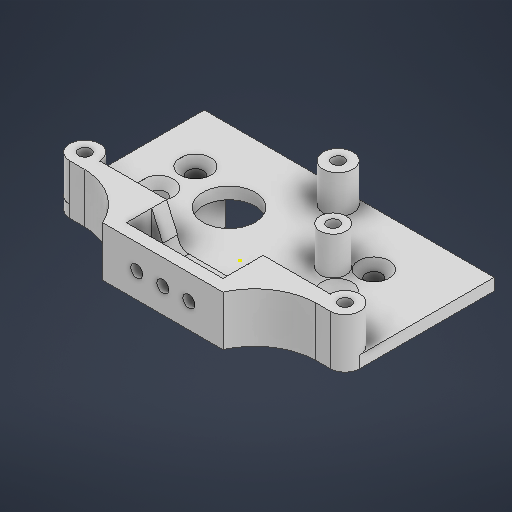
# Autodesk Inventor part: ПЕРЕДНИЙ ЗАХВАТ
Saved by Autodesk Inventor 2025 (Build 290162000, 162)
## iProperties
Created: 2025-02-17
Part Number: ПЕРЕДНИЙ ЗАХВАТ
Material: Типовые
Document SubType Name: Modeling
Designer: Phantom
Density: 1 g/cm^3
Appearance: По умолчанию
Author: Phantom
Autodesk Inventor part; units mm, degrees
ref_plane "YZ Plane" through (0, 0, 0) normal (1, 0, 0) x (0, 1, 0)
ref_plane "XZ Plane" through (0, 0, 0) normal (0, 1, 0) x (-1, 0, 0)
ref_plane "XY Plane" through (0, 0, 0) normal (0, 0, 1) x (1, 0, 0)
sketch "Эскиз1" plane through (0, 0, 0) normal (0, 1, 0) x (-1, 0, 0)
  line L0 (-30, 30.5) -> (30, 30.5)
  line L1 (30, 30.5) -> (30, -30.5)
  line L2 (30, -30.5) -> (-30, -30.5)
  line L3 (-30, -30.5) -> (-30, 30.5)
  line L4 (-30, 30.5) -> (30, 30.5) construction
  circle A0 centre (0, -26.5) radius 1.6
  circle A1 centre (-14, -11.15) radius 2.1
  circle A2 centre (14, -11.15) radius 7
  point P0 (0, 0)
  dimension "d0" = 60
  dimension "d2" = 61
  dimension "d3" = 30
  dimension "d4" = 3.2
  dimension "d5" = 4
  dimension "d6" = 4.2
  dimension "d7" = 19.35
  dimension "d8" = 28
  dimension "d9" = 14
  dimension "d11" = 19.35
  dimension "d13" = 16
  constraints: 10 end point, 3 centre point, 2 horizontal, 2 parallel, 1 collinear, 1 perpendicular
  measures "d0" distance of L0.start L0.end
  measures "d2" distance of L0.end L1.end
  measures "d3" distance from line of L3 A0.centre
  measures "d4" diameter of A0
  measures "d5" distance from line of L2 A0.centre
  measures "d6" diameter of A1
  measures "d7" distance from line of L2 A1.centre
  measures "d8" distance of A1.centre A2.centre
  measures "d9" diameter of A2
  measures "d11" distance from line of L2 A2.centre
  measures "d13" distance from line of L3 A1.centre
extrude "Выдавливание1" add sketch "Эскиз1" along normal blind 3.2
sketch "Эскиз2" plane through (0, 3.2, 0) normal (0, 1, 0) x (1, 0, 0)
  line L0 (30, 30.5) -> (-30, 30.5) projected
  line L1 (-30, 30.5) -> (-30, -5.65)
  line L2 (-30, 30.5) -> (-30, -30.5) projected
  line L3 (-30, -5.65) -> (30, -5.65)
  line L4 (-30, -5.65) -> (30, -5.65)
  line L5 (30, -5.65) -> (30, -9.65)
  line L6 (30, -9.65) -> (-30, -9.65)
  line L7 (-30, -9.65) -> (-30, -5.65)
  circle A0 centre (0, 26.5) radius 1.6 projected
  circle A1 centre (0, 26.5) radius 4
  line L8 (4, 26.5) -> (4, 30.5)
  line L9 (-4, 26.5) -> (-4, 30.5)
  point P0 (0, 0)
  dimension "d16" = 36.15
  dimension "d17" = 60
  dimension "d18" = 4
  dimension "d19" = 8
  constraints: 16 end point, 4 perpendicular, 3 point on line, 2 parallel, 2 point on circle, 2 tangent, 1 centre point, 1 coincident, 1 horizontal
  measures "d16" distance of L0.end L1.end
  measures "d17" distance of L5.end L6.end
  measures "d18" distance of L4.end L5.end
  measures "d19" diameter of A1
extrude "Выдавливание2" add sketch "Эскиз2" along normal blind 10.2 contours A1 | L3 L5 L6 L2
sketch "Эскиз3" plane through (0, 0, 0) normal (0, -1, 0) x (1, 0, 0)
  arc A0 (-23.679, -20.65) -> (-23.512, -21.65) centre (-22.7453, -21.008) ccw
  line L0 (-24.037, -20.65) -> (-24.037, -1.65)
  arc A1 (-23.512, -0.65) -> (-23.679, -1.65) centre (-22.7453, -1.292) ccw
  line L1 (17.25, -0.65) -> (-22.25, -0.65)
  arc A2 (16.988, -1.65) -> (15.988, -0.65) centre (15.988, -1.65) ccw
  line L2 (15.963, -20.65) -> (15.963, -1.65)
  arc A3 (15.988, -21.65) -> (16.988, -20.65) centre (15.988, -20.65) ccw
  line L3 (17.25, -21.65) -> (-22.25, -21.65)
  circle A4 centre (-28.037, -16.15) radius 2.1
  circle A5 centre (-28.037, -6.15) radius 2.1
  circle A6 centre (19.963, -6.15) radius 2.1
  circle A7 centre (19.963, -16.15) radius 2.1
  line L4 (2.4, 0.15) -> (9.6, 0.15)
  circle A8 centre (-14, -11.15) radius 7 projected
  line L5 (-28.037, -2.15) -> (-24.037, -2.15)
  line L6 (-28.037, -2.15) -> (-32.037, -2.15)
  line L7 (-32.037, -2.15) -> (-32.037, -20.15)
  line L8 (-32.037, -20.15) -> (-24.037, -20.15)
  line L9 (-2.5, -0.65) -> (-2.5, -38)
  line L10 (19.963, -2.15) -> (15.963, -2.15)
  line L11 (19.963, -2.15) -> (23.963, -2.15)
  line L12 (23.963, -2.15) -> (23.963, -20.15)
  line L13 (23.963, -20.15) -> (15.963, -20.15)
  line L14 (16.988, -20.65) -> (16.988, -20.15)
  line L15 (17.704, -2.15) -> (16.988, -1.65)
  line L16 (-30, -30.5) -> (-30, 30.5) projected
  point P0 (0, 0)
  point P1 (-14, -11.15)
  point P2 (24.738, -11.15)
  point P3 (-28.037, -6.15)
  point P4 (19.846, -6.15)
  point P5 (-28.037, -6.15)
  constraints: 32 end point, 8 centre point, 8 point on circle, 4 point on line, 2 perpendicular, 2 vertical, 1 coincident, 1 midpoint
extrude "Выдавливание3" add sketch "Эскиз3" along normal blind 11 contours L8 L16 A4 A5 L6 L5 L0 | L8 L7 L6 L16 A5 A4 | L10 L11 L12 L13 L2
sketch "Эскиз4" plane through (0, 0, 0) normal (0, 1, 0) x (1, 0, 0)
  line L0 (-30, 5.4039) -> (-30, 2.15) projected
  line L1 (-32.037, 20.15) -> (-30, 20.15) projected
  line L2 (-32.037, 2.15) -> (-32.037, 20.15) projected
  line L3 (-30, 2.15) -> (-32.037, 2.15) projected
  line L4 (30, -9.65) -> (-30, -9.65) projected
  line L5 (-30, -9.65) -> (-30, -30.5) projected
  line L6 (-30, -30.5) -> (30, -30.5) projected
  line L7 (30, -30.5) -> (30, -9.65) projected
  line L8 (-30, -30.5) -> (-31.25, -30.5)
  line L9 (-31.25, -30.5) -> (-31.25, 30.5)
  line L10 (-31.25, 30.5) -> (-30, 30.5)
  line L11 (-30, 30.5) -> (-30, -30.5)
  line L12 (30, 30.5) -> (-30, 30.5) projected
  line L13 (-30, 15.4039) -> (-30, 6.8961) projected
  arc A0 (-30, 16.8961) -> (-30, 15.4039) centre (-28.037, 16.15) ccw projected
  line L14 (-30, 20.15) -> (-30, 16.8961) projected
  arc A1 (-30, 6.8961) -> (-30, 5.4039) centre (-28.037, 6.15) ccw projected
  point P0 (0, 0)
  point P1 (-31.25, 20.15)
  point P2 (-31.25, 2.15)
  point P3 (-30, 2.15)
  point P4 (-30, 5.4039)
  point P5 (-30, 2.15)
  point P6 (-31.25, 2.15)
  point P7 (-31.25, 20.15)
  dimension "d25" = 0
  constraints: 8 end point, 2 parallel, 1 collinear, 1 horizontal, 1 perpendicular
  measures "d25" distance between parallel lines of L10 L12
extrude "Выдавливание4" add sketch "Эскиз4" along normal up to surface (3.2 mm away) contours A1 L11 | L0 L3 L9 L1 L11 A0 A1 | L11 L5 L8 L9 L3 | A0 L11 | L9 L10 L11 L1
sketch "Эскиз5" plane through (0, 3.2, 0) normal (0, 1, 0) x (1, 0, 0)
  circle A0 centre (14, 11.15) radius 2.1 projected
  circle A1 centre (-14, 11.15) radius 7 projected
  circle A2 centre (0, 26.5) radius 4 projected
  line L0 (30, -9.65) -> (-30, -9.65) projected
  line L1 (-30, -5.65) -> (-30, -9.65) projected
  line L2 (-30, -5.65) -> (30, -5.65) projected
  line L3 (30, -5.65) -> (30, 30.5) projected
  line L4 (30, 30.5) -> (0, 30.5) projected
  line L5 (-31.25, -30.5) -> (-31.25, 30.5) projected
  line L6 (30, -30.5) -> (-31.25, -30.5) projected
  line L7 (30, -30.5) -> (30, -9.65) projected
  line L8 (-30, -9.65) -> (-31.25, -9.65)
  line L9 (-31.25, -9.65) -> (-31.25, -5.65)
  line L10 (-31.25, -5.65) -> (-30, -5.65)
  line L11 (-30, -5.65) -> (-30, -9.65)
  line L12 (0, 30.5) -> (-31.25, 30.5) projected
  point P0 (0, 0)
  constraints: 8 end point, 2 parallel, 1 horizontal, 1 perpendicular, 1 point on line, 1 vertical alignment
extrude "Выдавливание5" add sketch "Эскиз5" along normal up to surface (10.2 mm away) contours L10 L1 L8 L5
sketch "Эскиз6" plane through (0, -11, 0) normal (0, -1, 0) x (1, 0, 0)
  point P0 (0, 0)
sketch "Эскиз7" plane through (0, -11, 0) normal (0, -1, 0) x (1, 0, 0)
  line L0 (15.963, -20.15) -> (15.963, -2.15) projected
  line L1 (15.963, -11.15) -> (23.963, -11.15)
  line L2 (23.963, -2.15) -> (23.963, -20.15) projected
  line L3 (15.963, -10.4) -> (23.963, -10.4)
  line L4 (23.963, -10.4) -> (23.963, -11.9)
  line L5 (23.963, -11.9) -> (15.963, -11.9)
  line L6 (15.963, -11.9) -> (15.963, -10.4)
  line L7 (15.963, -10.4) -> (23.963, -11.9) construction
  line L8 (23.963, -10.4) -> (15.963, -11.9) construction
  line L9 (-32.037, -20.15) -> (-24.037, -20.15) projected
  line L10 (15.963, -20.15) -> (-24.037, -20.15)
  line L11 (-4.037, -20.15) -> (-4.037, 5)
  line L12 (-24.037, -11.15) -> (-32.037, -11.15)
  line L13 (-24.037, -10.4) -> (-32.037, -10.4)
  line L14 (-32.037, -10.4) -> (-32.037, -11.9)
  line L15 (-32.037, -11.9) -> (-24.037, -11.9)
  line L16 (-24.037, -11.9) -> (-24.037, -10.4)
  line L17 (-24.037, -10.4) -> (-32.037, -11.9) construction
  line L18 (-32.037, -10.4) -> (-24.037, -11.9) construction
  point P0 (0, 0)
  point P1 (19.963, -11.15)
  point P2 (15.963, -11.9)
  point P3 (15.963, -10.4)
  point P4 (-28.037, -11.15)
  dimension "d30" = 8
  dimension "d31" = 1.5
  constraints: 32 end point, 7 symmetric about line, 6 midpoint, 2 horizontal, 2 parallel, 1 perpendicular, 1 vertical
  measures "d30" distance of L4.end L5.end
  measures "d31" distance of L3.end L4.end
extrude "Выдавливание6" cut sketch "Эскиз7" against normal blind 5
fillet "Сопряжение1" radius 1 4 edges at (19.963, -11, -11.9) (19.963, -11, -10.4) (-28.037, -11, -11.9) (-28.037, -11, -10.4)
sketch "Эскиз8" plane through (0, -11, 0) normal (0, -1, 0) x (1, 0, 0)
  circle A0 centre (-28.037, -6.15) radius 2.1 projected
  circle A1 centre (-28.037, -16.15) radius 2.1 projected
  circle A2 centre (19.963, -6.15) radius 2.1 projected
  circle A3 centre (19.963, -16.15) radius 2.1 projected
  point P0 (0, 0)
extrude "Выдавливание7" cut sketch "Эскиз8" against normal through all
sketch "Эскиз9" plane through (0, 3.2, 0) normal (0, 1, 0) x (1, 0, 0)
  line L0 (30, -9.65) -> (-31.25, -9.65) projected
  line L1 (-31.25, -30.5) -> (-31.25, -9.65) projected
  line L2 (30, -30.5) -> (-31.25, -30.5) projected
  line L3 (30, -30.5) -> (30, -9.65) projected
  point P0 (0, 0)
extrude "Выдавливание8" cut sketch "Эскиз9" against normal blind 10
sketch "Эскиз11" plane through (0, 3.2, 0) normal (0, 1, 0) x (1, 0, 0)
  circle A0 centre (14, 11.15) radius 2.1 projected
  circle A1 centre (-14, 11.15) radius 7 projected
  circle A2 centre (0, 26.5) radius 4 projected
  line L0 (-31.25, -5.65) -> (30, -5.65) projected
  line L1 (30, -5.65) -> (30, 30.5) projected
  line L2 (30, 30.5) -> (0, 30.5) projected
  circle A3 centre (14, 11.15) radius 3.5
  circle A4 centre (14, 11.15) radius 1.575
  line L3 (0, 30.5) -> (-31.25, 30.5) projected
  line L4 (-31.25, -5.65) -> (-31.25, 30.5) projected
  point P0 (0, 0)
  dimension "d49" = 7
  dimension "d50" = 3.15
  constraints: 2 centre point, 2 coincident, 1 vertical alignment
  measures "d49" diameter of A3
  measures "d50" diameter of A4
extrude "Выдавливание10" add sketch "Эскиз11" along normal up to surface (10.2 mm away) contours A0 | A3
sketch "Эскиз12" plane through (14, 3.2, -11.15) normal (0, -1, 0) x (1, 0, 0)
  circle A0 centre (0, 0) radius 1.575 projected
  circle A1 centre (0, 0) radius 2.1 projected
  point P0 (-14, 11.15)
sketch "Эскиз13" plane through (0, 13.4, 0) normal (0, 1, 0) x (1, 0, 0)
  line L0 (-31.25, -9.65) -> (-31.25, 30.5) projected
  line L1 (30, -9.65) -> (-31.25, -9.65)
  line L2 (-31.25, -9.65) -> (-31.25, 30.5)
  line L3 (-31.25, 30.5) -> (30, 30.5)
  line L4 (30, 30.5) -> (30, -9.65)
  circle A0 centre (0, 26.5) radius 1.6 projected
  circle A1 centre (0, 26.5) radius 4 projected
  circle A2 centre (0, 26.5) radius 1.6 projected
  circle A3 centre (0, -3.55) radius 1.6
  circle A4 centre (0, -3.55) radius 4
  circle A5 centre (0, -3.55) radius 1.6
  line L5 (4, -3.55) -> (4, -8.05)
  line L6 (-31.25, -5.65) -> (30, -5.65) projected
  circle A6 centre (14, 11.15) radius 3.5 projected
  circle A7 centre (-14, 11.15) radius 7 projected
  circle A8 centre (0, 26.5) radius 4 projected
  line L7 (-31.25, -5.65) -> (30, -5.65) projected
  line L8 (30, -5.65) -> (30, 30.5) projected
  line L9 (30, 30.5) -> (0, 30.5) projected
  line L10 (-4, -3.55) -> (-4, -8.05)
  line L11 (0, 30.5) -> (-31.25, 30.5) projected
  line L12 (-31.25, -5.65) -> (-31.25, 30.5) projected
  point P0 (0, 0)
  point P1 (-30.775, 25.15)
  point P2 (0, -1.15)
  point P3 (-4, -5.65)
  point P4 (0, -3.15)
  point P5 (3.4044, -5.65)
  point P6 (4, -5.65)
  point P7 (-3.4044, -5.65)
  dimension "d65" = 3.2
  dimension "d66" = 3.2
  dimension "d67" = 8
  constraints: 12 end point, 3 centre point, 2 parallel, 2 perpendicular, 2 point on circle, 1 horizontal, 1 tangent, 1 vertical, 1 vertical alignment, 1 other
  measures "d65" diameter of A3
  measures "d66" diameter of A5
  measures "d67" diameter of A4
extrude "Выдавливание12" add sketch "Эскиз13" against normal up to surface (10.2 mm away) contours L10 A4 L6 | A4 L6 | L6 A4 L5 picked at (-0.0643, -5.4794)
sketch "Эскиз14" plane through (0, 3.2, 0) normal (0, 1, 0) x (1, 0, 0)
  circle A0 centre (0, -3.55) radius 1.6 projected
  point P0 (0, 0)
extrude "Выдавливание13" cut sketch "Эскиз14" against normal blind 10
sketch "Эскиз16" plane through (0, 3.2, 0) normal (0, 1, 0) x (1, 0, 0)
  point P0 (0, 0)
sketch "Эскиз19" plane through (0, 3.2, 0) normal (0, 1, 0) x (1, 0, 0)
  line L0 (-31.25, 2.15) -> (-31.25, 20.15) projected
  line L1 (-32.037, 20.15) -> (-31.25, 20.15) projected
  line L2 (-32.037, 2.15) -> (-32.037, 20.15) projected
  line L3 (-31.25, 2.15) -> (-32.037, 2.15) projected
  line L4 (-31.25, 2.15) -> (-31.25, -9.65) projected
  line L5 (-31.25, -9.65) -> (-32.037, -9.65)
  line L6 (-32.037, -9.65) -> (-32.037, 30.5)
  line L7 (-32.037, 30.5) -> (-31.25, 30.5)
  line L8 (-31.25, 30.5) -> (-31.25, -9.65)
  point P0 (0, 0)
  constraints: 8 end point, 2 parallel, 1 horizontal, 1 perpendicular
extrude "Выдавливание17" add sketch "Эскиз19" against normal up to surface (3.2 mm away)
fillet "Сопряжение4" radius 5 4 edges at (-28.037, 0, -20.15) (19.963, 0, -20.15) (19.963, 0, -2.15) (-28.037, 0, -2.15)
sketch "Эскиз20" plane through (0, -11, 0) normal (0, -1, 0) x (1, 0, 0)
  circle A0 centre (-14, -11.15) radius 7 projected
  circle A1 centre (0, -26.5) radius 1.6 projected
  circle A2 centre (0, 3.55) radius 1.6 projected
  line L0 (-24.037, 2.85) -> (-32.037, 2.85) projected
  line L1 (-24.037, 2.85) -> (-24.037, -25.15) projected
  line L2 (-32.037, -25.15) -> (-24.037, -25.15) projected
  line L3 (-32.037, -25.15) -> (-32.037, -30.5) projected
  line L4 (30, -30.5) -> (-32.037, -30.5) projected
  line L5 (30, 9.65) -> (30, -30.5) projected
  line L6 (30, 9.65) -> (-32.037, 9.65) projected
  line L7 (-32.037, 9.65) -> (-32.037, 2.85) projected
  line L8 (23.963, 2.85) -> (23.963, -25.15) projected
  line L9 (15.963, -25.15) -> (23.963, -25.15) projected
  line L10 (15.963, -25.15) -> (15.963, -11.8961) projected
  arc A3 (15.963, -10.4039) -> (15.963, -11.8961) centre (14, -11.15) ccw projected
  line L11 (15.963, -10.4039) -> (15.963, 2.85) projected
  line L12 (23.963, 2.85) -> (15.963, 2.85) projected
  circle A4 centre (14, -11.15) radius 3.5
  point P0 (0, 0)
  dimension "d83" = 7
  constraints: 1 centre point, 1 coincident
  measures "d83" diameter of A4
extrude "Выдавливание18" cut sketch "Эскиз20" against normal up to surface (11 mm away) contours A4 L10 A3 L11 | L11 A3 L10 A4
chamfer "Фаска4" distance 2 angle 45 5 edges at (17.863, 3.2, -6.15) (17.863, 3.2, -16.15) (-30.137, 3.2, -6.15) (-30.137, 3.2, -16.15) (16.1, 0, -11.15)
sketch "Эскиз21" plane through (0, 3.2, 0) normal (0, 1, 0) x (1, 0, 0)
  circle A0 centre (19.963, 6.15) radius 4.1 projected
  arc A1 (-32.037, 15.25) -> (-32.037, 17.05) centre (-28.037, 16.15) ccw projected
  line L0 (-32.037, 15.25) -> (-32.037, 7.05) projected
  arc A2 (-32.037, 5.25) -> (-32.037, 7.05) centre (-28.037, 6.15) ccw projected
  line L1 (-32.037, 5.25) -> (-32.037, -9.65) projected
  line L2 (-32.037, -9.65) -> (-31.25, -9.65) projected
  line L3 (-31.25, -5.65) -> (-31.25, -9.65) projected
  line L4 (-31.25, -5.65) -> (-4, -5.65) projected
  line L5 (-4, -5.65) -> (-4, -3.55) projected
  arc A3 (4, -3.55) -> (-4, -3.55) centre (0, -3.55) ccw projected
  line L6 (4, -3.55) -> (4, -5.65) projected
  line L7 (4, -5.65) -> (30, -5.65) projected
  line L8 (30, -5.65) -> (30, 30.5) projected
  line L9 (30, 30.5) -> (0, 30.5) projected
  circle A4 centre (0, 26.5) radius 4 projected
  line L10 (0, 30.5) -> (-32.037, 30.5) projected
  line L11 (-32.037, 30.5) -> (-32.037, 17.05) projected
  circle A5 centre (-14, 11.15) radius 7 projected
  circle A6 centre (14, 11.15) radius 3.5 projected
  circle A7 centre (19.963, 16.15) radius 4.1 projected
  line L12 (-32.037, -9.65) -> (-31.25, -9.65)
  line L13 (-31.25, -9.65) -> (-31.25, -5.65)
  line L14 (-31.25, -5.65) -> (-32.037, -5.65)
  line L15 (-32.037, -5.65) -> (-32.037, -9.65)
  point P0 (0, 0)
  constraints: 8 end point, 2 parallel, 1 horizontal, 1 perpendicular, 1 vertical alignment
extrude "Выдавливание19" add sketch "Эскиз21" along normal up to surface (10.2 mm away) contours L14 L3 L2 L1
sketch "Эскиз22" plane through (30, 0, 9.65) normal (0, 0, 1) x (1, 0, 0)
  point P0 (-30, 0)
sketch "Эскиз23" plane through (30, 0, 9.65) normal (0, 0, 1) x (1, 0, 0)
  line L0 (0, 13.4) -> (0, 0) projected
  line L1 (0, 6.7) -> (-62.037, 6.7)
  line L2 (-62.037, 3.2) -> (-62.037, 13.4) projected
  circle A0 centre (-31.0185, 6.7) radius 11
  line L3 (-42.0185, 6.7) -> (-44.0185, 6.7)
  line L4 (-20.0185, 6.7) -> (-18.0185, 6.7)
  line L5 (0, 13.4) -> (-62.037, 13.4) projected
  line L6 (-44.0185, 6.7) -> (-47.2185, 6.7)
  line L7 (-47.2185, 6.7) -> (-47.2185, 13.4)
  line L8 (-47.2185, 13.4) -> (-44.0185, 13.4)
  line L9 (-44.0185, 13.4) -> (-44.0185, 6.7)
  line L10 (-44.0185, 6.7) -> (-47.2185, 6.7)
  line L11 (-47.2185, 6.7) -> (-47.2185, 0)
  line L12 (-47.2185, 0) -> (-44.0185, 0)
  line L13 (-44.0185, 0) -> (-44.0185, 6.7)
  line L14 (-31.0185, 17.7) -> (-31.0185, -4.3)
  line L15 (-20.0185, 6.7) -> (-18.0185, 6.7)
  line L16 (-18.0185, 6.7) -> (-14.8185, 6.7)
  line L17 (-14.8185, 6.7) -> (-14.8185, 13.4)
  line L18 (-14.8185, 13.4) -> (-18.0185, 13.4)
  line L19 (-18.0185, 13.4) -> (-18.0185, 6.7)
  line L20 (-18.0185, 6.7) -> (-14.8185, 6.7)
  line L21 (-14.8185, 6.7) -> (-14.8185, 0)
  line L22 (-14.8185, 0) -> (-18.0185, 0)
  line L23 (-18.0185, 0) -> (-18.0185, 6.7)
  point P0 (-30, 0)
  dimension "d91" = 22
  dimension "d92" = 2
  dimension "d93" = 2
  dimension "d94" = 3.2
  constraints: 42 end point, 8 point on line, 6 symmetric about line, 4 parallel, 4 point on circle, 3 horizontal, 2 midpoint, 2 perpendicular, 1 centre point
  measures "d91" diameter of A0
  measures "d92" distance of L3.start L3.end
  measures "d93" distance of L4.start L4.end
  measures "d94" distance of L7.end L8.end
extrude "Выдавливание20" add sketch "Эскиз23" along normal blind 10 contours L17 L1 L19 L5 | L21 L22 L23 L1 | L9 L1 L7 L5 | L13 L12 L11 L1
sketch "Эскиз24" plane through (30, 0, 19.65) normal (0, 0, 1) x (1, 0, 0)
  line L0 (-44.0185, 13.4) -> (-47.2185, 13.4) projected
  line L1 (-47.2185, 13.4) -> (-47.2185, 0) projected
  line L2 (-47.2185, 0) -> (-44.0185, 0) projected
  line L3 (-44.0185, 0) -> (-44.0185, 13.4) projected
  line L4 (-14.8185, 13.4) -> (-18.0185, 13.4) projected
  line L5 (-18.0185, 13.4) -> (-18.0185, 0) projected
  line L6 (-18.0185, 0) -> (-14.8185, 0) projected
  line L7 (-14.8185, 0) -> (-14.8185, 13.4) projected
  line L8 (-14.8185, 0) -> (-47.2185, 0)
  line L9 (-47.2185, 0) -> (-47.2185, 13.4)
  line L10 (-47.2185, 13.4) -> (-14.8185, 13.4)
  line L11 (-14.8185, 13.4) -> (-14.8185, 0)
  line L12 (-47.2185, 6.7) -> (-14.8185, 6.7)
  line L13 (-31.0185, 6.7) -> (-38.0185, 6.7)
  circle A0 centre (-38.0185, 6.7) radius 1.6
  line L14 (-31.0185, 6.7) -> (-31.0185, 13)
  circle A1 centre (-24.0185, 6.7) radius 1.6
  line L15 (-47.2185, 0) -> (-14.8185, 0)
  line L16 (-14.8185, 0) -> (-14.8185, 13.4)
  line L17 (-14.8185, 13.4) -> (-47.2185, 13.4)
  line L18 (-47.2185, 13.4) -> (-47.2185, 0)
  point P0 (-30, 0)
  dimension "d97" = 7
  dimension "d98" = 3.2
  constraints: 22 end point, 4 parallel, 3 midpoint, 2 centre point, 2 horizontal, 2 perpendicular, 1 coincident, 1 point on line, 1 symmetric about line, 1 vertical, 1 other
  measures "d97" distance of L13.start L13.end
  measures "d98" diameter of A0
extrude "Выдавливание21" add sketch "Эскиз24" against normal blind 3.2 contours L10 L5 L12 A1 A0 L3 | L12 A0 A1 L5 L8 L3
fillet "Сопряжение5" radius 17 2 edges at (-17.2185, 6.7, 9.65) (15.1815, 6.7, 9.65)
sketch "Эскиз26" plane through (0, 13.4, 0) normal (0, 1, 0) x (1, 0, 0)
  line L0 (-14.0185, -9.65) -> (-14.0185, -16.45) projected
  line L1 (11.9815, -9.65) -> (-14.0185, -9.65) projected
  line L2 (11.9815, -9.65) -> (11.9815, -16.45) projected
  line L3 (-14.0185, -16.45) -> (11.9815, -16.45) projected
  circle A0 centre (0, -3.55) radius 1.6 projected
  line L4 (15.1815, -19.65) -> (-17.2185, -19.65) projected
  arc A1 (30, -9.65) -> (15.1815, -19.65) centre (30.6796, -26.6364) ccw projected
  line L5 (30, -9.65) -> (30, -5.65) projected
  line L6 (30, -5.65) -> (4, -5.65) projected
  line L7 (4, -5.65) -> (4, -3.55) projected
  arc A2 (4, -3.55) -> (-4, -3.55) centre (0, -3.55) ccw projected
  line L8 (-4, -3.55) -> (-4, -5.65) projected
  line L9 (-4, -5.65) -> (-32.037, -5.65) projected
  line L10 (-32.037, -9.65) -> (-32.037, -5.65) projected
  arc A3 (-17.2185, -19.65) -> (-32.037, -9.65) centre (-32.7166, -26.6364) ccw projected
  line L11 (4, -5.65) -> (-4, -5.65)
  point P0 (0, 0)
  constraints: 2 end point, 1 collinear
extrude "Выдавливание22" cut sketch "Эскиз26" against normal up to surface (10.2 mm away) contours L11 L8 A2 L7
sketch "Эскиз27" plane through (30, 3.2, 5.65) normal (0, 0, -1) x (-1, 0, 0)
  circle A0 centre (38.0185, 3.5) radius 1.6 projected
  circle A1 centre (24.0185, 3.5) radius 1.6 projected
  line L0 (24.0185, 3.5) -> (38.0185, 3.5)
  line L1 (31.0185, 3.5) -> (24.0185, 3.5)
  circle A2 centre (24.0185, 3.5) radius 3
  line L2 (24.0185, 3.5) -> (38.0185, 3.5)
  circle A3 centre (38.0185, 3.5) radius 3
  circle A4 centre (31.0185, 3.5) radius 3
  line L3 (24.0185, 6.5) -> (38.0185, 6.5)
  line L4 (24.0185, 0.5) -> (38.0185, 0.5)
  point P0 (30, -3.2)
  dimension "d108" = 7
  dimension "d109" = 6
  dimension "d110" = 14
  dimension "d111" = 6
  dimension "d112" = 6
  constraints: 10 end point, 5 coincident, 4 point on circle, 3 centre point, 2 point on line, 2 tangent, 1 horizontal, 1 midpoint
  measures "d108" distance of L1.start L1.end
  measures "d109" diameter of A2
  measures "d110" distance of L2.start L2.end
  measures "d111" diameter of A3
  measures "d112" diameter of A4
extrude "Выдавливание23" cut sketch "Эскиз27" against normal up to surface (10.8 mm away) contours A0 | A1 | L0 A4 | L0 A4 | A4 L3 A3 L0 | L0 A3 L4 A4 | A4 L4 A2 L0 | L0 A2 L3 A4 | A3 | A2
sketch "Эскиз28" plane through (30, 0, 19.65) normal (0, 0, 1) x (1, 0, 0)
  circle A0 centre (-38.0185, 6.7) radius 1.6 projected
  circle A1 centre (-24.0185, 6.7) radius 1.6 projected
  line L0 (-14.8185, 13.4) -> (-47.2185, 13.4) projected
  line L1 (-47.2185, 13.4) -> (-47.2185, 0) projected
  line L2 (-47.2185, 0) -> (-14.8185, 0) projected
  line L3 (-14.8185, 0) -> (-14.8185, 13.4) projected
  line L4 (-38.0185, 6.7) -> (-24.0185, 6.7)
  circle A2 centre (-31.0185, 6.7) radius 1.6
  point P0 (-30, 0)
  constraints: 2 end point, 1 centre point, 1 horizontal, 1 midpoint
extrude "Выдавливание24" cut sketch "Эскиз28" against normal blind 10 contours A2 L4 | L4 A2
sketch "Эскиз29" plane through (0, 3.2, 0) normal (0, 1, 0) x (1, 0, 0)
  circle A0 centre (0, -3.55) radius 1.6 projected
  line L0 (-32.037, -5.65) -> (30, -5.65) projected
  line L1 (30, -5.65) -> (30, 30.5) projected
  line L2 (30, 30.5) -> (0, 30.5) projected
  circle A1 centre (0, 26.5) radius 4 projected
  line L3 (0, 30.5) -> (-32.037, 30.5) projected
  line L4 (-32.037, 30.5) -> (-32.037, 17.05) projected
  arc A2 (-32.037, 15.25) -> (-32.037, 17.05) centre (-28.037, 16.15) ccw projected
  line L5 (-32.037, 15.25) -> (-32.037, 7.05) projected
  arc A3 (-32.037, 5.25) -> (-32.037, 7.05) centre (-28.037, 6.15) ccw projected
  line L6 (-32.037, 5.25) -> (-32.037, -5.65) projected
  circle A4 centre (19.963, 6.15) radius 4.1 projected
  circle A5 centre (-14, 11.15) radius 7 projected
  circle A6 centre (14, 11.15) radius 3.5 projected
  circle A7 centre (19.963, 16.15) radius 4.1 projected
  point P0 (0, 0)
  constraints: 1 vertical alignment
extrude "Выдавливание25" add sketch "Эскиз29" against normal up to surface (3.2 mm away) contours A0
sketch "Эскиз30" plane through (0, 3.2, 0) normal (0, 1, 0) x (1, 0, 0)
  line L0 (-32.037, -5.65) -> (30, -5.65) projected
  line L1 (30, -5.65) -> (30, 30.5) projected
  line L2 (30, 30.5) -> (0, 30.5) projected
  circle A0 centre (0, 26.5) radius 4 projected
  line L3 (0, 30.5) -> (-32.037, 30.5) projected
  line L4 (-32.037, 30.5) -> (-32.037, 17.05) projected
  arc A1 (-32.037, 15.25) -> (-32.037, 17.05) centre (-28.037, 16.15) ccw projected
  line L5 (-32.037, 15.25) -> (-32.037, 7.05) projected
  arc A2 (-32.037, 5.25) -> (-32.037, 7.05) centre (-28.037, 6.15) ccw projected
  line L6 (-32.037, 5.25) -> (-32.037, -5.65) projected
  circle A3 centre (19.963, 6.15) radius 4.1 projected
  circle A4 centre (-14, 11.15) radius 7 projected
  circle A5 centre (14, 11.15) radius 3.5 projected
  circle A6 centre (19.963, 16.15) radius 4.1 projected
  line L7 (-32.037, 30.5) -> (-38.037, 30.5)
  line L8 (-38.037, 30.5) -> (-38.037, -5.65)
  line L9 (-38.037, -5.65) -> (-32.037, -5.65)
  line L10 (-32.037, -5.65) -> (-32.037, 30.5)
  line L11 (30, 30.5) -> (36, 30.5)
  line L12 (36, 30.5) -> (36, -5.65)
  line L13 (36, -5.65) -> (30, -5.65)
  line L14 (30, -5.65) -> (30, 30.5)
  point P0 (0, 0)
  point P1 (-24.037, 25.15)
  dimension "d117" = 6
  dimension "d121" = 6
  constraints: 16 end point, 4 parallel, 2 horizontal, 2 perpendicular, 1 vertical alignment
  measures "d117" distance of L9.end L8.end
  measures "d121" distance of L12.end L13.end
extrude "Выдавливание26" add sketch "Эскиз30" against normal up to surface (3.2 mm away) contours L9 L8 L7 L4 L10 L5 L6 | L1 L11 L12 L13
sketch "Эскиз31" plane through (0, 3.2, 0) normal (0, 1, 0) x (1, 0, 0)
  line L0 (-38.037, -5.65) -> (-32.037, -5.65) projected
  line L1 (-38.037, -5.65) -> (-33.537, -5.65)
  circle A0 centre (-36.037, -5.65) radius 1.6
  circle A1 centre (0, 26.5) radius 4 projected
  circle A2 centre (-36.037, -5.65) radius 4
  line L2 (30, -5.65) -> (36, -5.65) projected
  circle A3 centre (34, -5.65) radius 1.6
  circle A4 centre (34, -5.65) radius 4
  line L3 (-32.037, -9.65) -> (-32.037, -5.65) projected
  line L4 (-32.037, -5.65) -> (-36.037, -5.65)
  line L5 (30, -5.65) -> (34, -5.65)
  point P0 (0, 0)
  dimension "d124" = 3.2
  dimension "d125" = 8
  dimension "d128" = 3.2
  dimension "d129" = 8
  dimension "d132" = 4
  dimension "d133" = 4
  constraints: 6 end point, 4 centre point, 3 point on line, 2 coincident
  measures "d124" diameter of A0
  measures "d125" diameter of A2
  measures "d128" diameter of A3
  measures "d129" diameter of A4
  measures "d132" distance of L0.end L4.end
  measures "d133" distance of L2.start L5.end
extrude "Выдавливание27" add sketch "Эскиз31" along normal up to surface (10.2 mm away) contours A2 | A4
sketch "Эскиз32" plane through (0, 0, 0) normal (0, -1, 0) x (1, 0, 0)
  line L0 (-24.037, 2.85) -> (-32.037, 2.85) projected
  line L1 (-24.037, 2.85) -> (-24.037, -25.15) projected
  line L2 (-32.037, -25.15) -> (-24.037, -25.15) projected
  line L3 (-32.037, 2.85) -> (-32.037, -25.15) projected
  line L4 (-32.037, 5.65) -> (-38.037, 5.65) projected
  line L5 (-38.037, 5.65) -> (-38.037, -30.5) projected
  line L6 (36, -30.5) -> (-38.037, -30.5) projected
  line L7 (36, -30.5) -> (36, 5.65) projected
  line L8 (36, 5.65) -> (30, 5.65) projected
  line L9 (30, 9.65) -> (30, 5.65) projected
  arc A0 (15.1815, 19.65) -> (30, 9.65) centre (30.6796, 26.6364) ccw projected
  line L10 (-17.2185, 19.65) -> (15.1815, 19.65) projected
  arc A1 (-32.037, 9.65) -> (-17.2185, 19.65) centre (-32.7166, 26.6364) ccw projected
  line L11 (-32.037, 9.65) -> (-32.037, 5.65) projected
  arc A2 (15.963, -7.5505) -> (15.963, -14.7495) centre (14, -11.15) ccw projected
  line L12 (15.963, -7.5505) -> (15.963, 2.85) projected
  line L13 (23.963, 2.85) -> (15.963, 2.85) projected
  line L14 (23.963, 2.85) -> (23.963, -25.15) projected
  line L15 (15.963, -25.15) -> (23.963, -25.15) projected
  line L16 (15.963, -25.15) -> (15.963, -14.7495) projected
  circle A3 centre (-14, -11.15) radius 7 projected
  circle A4 centre (0, -26.5) radius 1.6 projected
  line L17 (11.9815, 16.45) -> (-14.0185, 16.45) projected
  line L18 (11.9815, 9.65) -> (11.9815, 16.45) projected
  line L19 (11.9815, 9.65) -> (-14.0185, 9.65) projected
  line L20 (-14.0185, 9.65) -> (-14.0185, 16.45) projected
  line L21 (-38.037, 2.1859) -> (-38.037, 5.65) projected
  line L22 (-38.037, 5.65) -> (-37.637, 5.65) projected
  arc A5 (-34.437, 5.65) -> (-37.637, 5.65) centre (-36.037, 5.65) ccw projected
  line L23 (-34.437, 5.65) -> (-32.037, 5.65) projected
  arc A6 (-32.037, 5.65) -> (-38.037, 2.1859) centre (-36.037, 5.65) ccw projected
  line L24 (35.6, 5.65) -> (36, 5.65) projected
  line L25 (36, 5.65) -> (36, 2.1859) projected
  arc A7 (36, 2.1859) -> (30, 5.65) centre (34, 5.65) ccw projected
  line L26 (30, 5.65) -> (32.4, 5.65) projected
  arc A8 (35.6, 5.65) -> (32.4, 5.65) centre (34, 5.65) ccw projected
  line L27 (-32.037, 9.65) -> (-40, 9.65)
  line L28 (-40, 9.65) -> (-40, -30.5)
  line L29 (-40, -30.5) -> (-38.037, -30.5)
  line L30 (30, 9.65) -> (38, 9.65)
  line L31 (38, 9.65) -> (38, -30.5)
  line L32 (38, -30.5) -> (36, -30.5)
  point P0 (0, 0)
  constraints: 12 end point, 5 perpendicular, 3 point on line
extrude "Выдавливание28" add sketch "Эскиз32" against normal up to surface (3.2 mm away) contours A6 L27 L11 | L4 A5 L5 A6 L28 | A6 L28 L27 | A6 L5 L29 L28 | L30 A7 L9 | A7 L7 L8 A8 | L30 L31 A7 | L7 A7 L31 L32
sketch "Эскиз33" plane through (0, 0, 0) normal (0, -1, 0) x (1, 0, 0)
  line L0 (35.6, 5.65) -> (32.4, 5.65) projected
  arc A0 (35.6, 5.65) -> (32.4, 5.65) centre (34, 5.65) ccw projected
  line L1 (-40, -30.5) -> (38, -30.5) projected
  line L2 (38, -30.5) -> (38, 9.65) projected
  line L3 (38, 9.65) -> (30, 9.65) projected
  arc A1 (15.1815, 19.65) -> (30, 9.65) centre (30.6796, 26.6364) ccw projected
  line L4 (-17.2185, 19.65) -> (15.1815, 19.65) projected
  arc A2 (-32.037, 9.65) -> (-17.2185, 19.65) centre (-32.7166, 26.6364) ccw projected
  line L5 (-32.037, 9.65) -> (-40, 9.65) projected
  line L6 (-40, 9.65) -> (-40, -30.5) projected
  line L7 (-24.037, 2.85) -> (-32.037, 2.85) projected
  line L8 (-24.037, 2.85) -> (-24.037, -25.15) projected
  line L9 (-32.037, -25.15) -> (-24.037, -25.15) projected
  line L10 (-32.037, 2.85) -> (-32.037, -25.15) projected
  arc A3 (-34.437, 5.65) -> (-37.637, 5.65) centre (-36.037, 5.65) ccw projected
  line L11 (-34.437, 5.65) -> (-37.637, 5.65) projected
  arc A4 (15.963, -7.5505) -> (15.963, -14.7495) centre (14, -11.15) ccw projected
  line L12 (15.963, -7.5505) -> (15.963, 2.85) projected
  line L13 (23.963, 2.85) -> (15.963, 2.85) projected
  line L14 (23.963, 2.85) -> (23.963, -25.15) projected
  line L15 (15.963, -25.15) -> (23.963, -25.15) projected
  line L16 (15.963, -25.15) -> (15.963, -14.7495) projected
  circle A5 centre (-14, -11.15) radius 7 projected
  circle A6 centre (0, -26.5) radius 1.6 projected
  line L17 (11.9815, 16.45) -> (-14.0185, 16.45) projected
  line L18 (11.9815, 9.65) -> (11.9815, 16.45) projected
  line L19 (11.9815, 9.65) -> (-14.0185, 9.65) projected
  line L20 (-14.0185, 9.65) -> (-14.0185, 16.45) projected
  circle A7 centre (-36.037, 5.65) radius 1.6
  circle A8 centre (34, 5.65) radius 1.6
  point P0 (0, 0)
  point P1 (-37.637, 5.65)
  constraints: 2 centre point, 2 coincident
extrude "Выдавливание29" cut sketch "Эскиз33" against normal through all contours A8 L0 | L0 A0 | L11 A3 | A7 L11
fillet "Сопряжение6" radius 4 2 edges at (-40, 1.6, 9.65) (38, 1.6, 9.65)
sketch "Эскиз34" plane through (0, 13.4, 0) normal (0, 1, 0) x (1, 0, 0)
  line L0 (30, -5.65) -> (-32.037, -5.65) projected
  line L1 (-32.037, -9.65) -> (-32.037, -5.65) projected
  arc A0 (-17.2185, -19.65) -> (-32.037, -9.65) centre (-32.7166, -26.6364) ccw projected
  line L2 (15.1815, -19.65) -> (-17.2185, -19.65) projected
  arc A1 (30, -9.65) -> (15.1815, -19.65) centre (30.6796, -26.6364) ccw projected
  line L3 (30, -9.65) -> (30, -5.65) projected
  line L4 (-14.0185, -9.65) -> (-14.0185, -16.45) projected
  line L5 (11.9815, -9.65) -> (-14.0185, -9.65) projected
  line L6 (11.9815, -9.65) -> (11.9815, -16.45) projected
  line L7 (-14.0185, -16.45) -> (11.9815, -16.45) projected
  circle A2 centre (-36.037, -5.65) radius 4 projected
  line L8 (-32.037, -9.65) -> (-36, -9.65) projected
  circle A3 centre (34, -5.65) radius 1.6 projected
  circle A4 centre (34, -5.65) radius 4 projected
  line L9 (34, -9.65) -> (30, -9.65) projected
  line L10 (30, -5.65) -> (-32.037, -5.65) projected
  line L11 (-32.037, -9.65) -> (-32.037, -5.65) projected
  arc A5 (-17.2185, -19.65) -> (-32.037, -9.65) centre (-32.7166, -26.6364) ccw projected
  line L12 (15.1815, -19.65) -> (-17.2185, -19.65) projected
  arc A6 (30, -9.65) -> (15.1815, -19.65) centre (30.6796, -26.6364) ccw projected
  line L13 (30, -9.65) -> (30, -5.65) projected
  line L14 (-14.0185, -9.65) -> (-14.0185, -16.45) projected
  line L15 (11.9815, -9.65) -> (-14.0185, -9.65) projected
  line L16 (11.9815, -9.65) -> (11.9815, -16.45) projected
  line L17 (-14.0185, -16.45) -> (11.9815, -16.45) projected
  circle A7 centre (-36.037, -5.65) radius 4 projected
  circle A8 centre (-36.037, -5.65) radius 1.6 projected
  arc A9 (-36.0185, -9.65) -> (-36, -9.65) centre (-36, -5.65) ccw projected
  line L18 (-32.037, -9.65) -> (-36, -9.65) projected
  line L19 (-32.037, -5.65) -> (-32.037, -9.65) projected
  arc A10 (-36.0185, -9.65) -> (-32.037, -5.65) centre (-36.037, -5.65) ccw projected
  point P0 (0, 0)
  point P1 (-36.0185, -9.65)
  constraints: 1 horizontal alignment, 1 other
extrude "Выдавливание30" add sketch "Эскиз34" against normal up to surface (10.2 mm away) contours A4 L9 L3 | L1 L8 A2
sketch "Эскиз35" plane through (30, 3.2, 5.65) normal (0, 0, -1) x (-1, 0, 0)
  arc A0 (38.0185, 0.5) -> (38.0185, 6.5) centre (38.0185, 3.5) ccw projected
  line L0 (38.0185, 0.5) -> (24.0185, 0.5) projected
  arc A1 (24.0185, 6.5) -> (24.0185, 0.5) centre (24.0185, 3.5) ccw projected
  line L1 (24.0185, 6.5) -> (38.0185, 6.5) projected
  line L2 (62.037, 0) -> (0, 0) projected
  line L3 (62.037, 0) -> (62.037, 10.2) projected
  line L4 (0, 10.2) -> (62.037, 10.2) projected
  line L5 (0, 0) -> (0, 10.2) projected
  line L6 (18.0185, 10.2) -> (44.0185, 10.2) projected
  line L7 (18.0185, -3.2) -> (18.0185, 10.2) projected
  line L8 (18.0185, 10.2) -> (21.0185, 3.5)
  arc A2 (24.0185, 6.5) -> (24.0185, 0.5) centre (24.0185, 3.5) ccw projected
  line L9 (44.0185, 10.2) -> (41.0185, 3.5)
  point P0 (30, -3.2)
  constraints: 4 end point, 3 point on circle
extrude "Выдавливание31" cut sketch "Эскиз35" against normal up to surface (10.8 mm away) contours A0 L1 A1 L8 L4 L9
